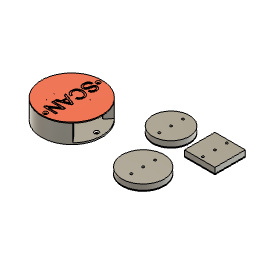
RFID Scanner und Tags (Autodesk Fusion 360 design; units mm, degrees)
Autodesk Fusion 360 part; units mm, degrees
sketch "Skizze1" plane through (0, 0, 0) normal (0, 1, 0) x (1, 0, 0)
  circle A0 centre (43.7248, 41.0876) radius 0.4571
  line L0 (55.1328, 36.6645) -> (55.1937, 36.6061)
  circle A1 centre (43.7248, 48.7056) radius 0.4571
  circle A2 centre (38.6462, 41.0876) radius 0.4571
  circle A3 centre (51.3428, 41.0876) radius 0.4571
  circle A4 centre (53.8821, 48.7056) radius 0.4571
  line L1 (7.4561, 1.7442) -> (7.4561, 59.7525) construction
  line L2 (55.1937, 36.6061) -> (55.2521, 36.6645)
  circle A5 centre (33.8119, 10.4896) radius 0.4571
  circle A6 centre (31.2827, -2.334) radius 0.4571
  circle A7 centre (53.3748, -5.0003) radius 0.4571
  circle A8 centre (20.871, 41.0876) radius 0.4571
  circle A9 centre (53.3748, -2.461) radius 0.4571
  circle A10 centre (47.6614, 7.5694) radius 2.5393
  line L3 (67.4454, 59.7662) -> (7.4454, 59.7754)
  circle A11 centre (48.8035, 18.2338) radius 0.4571
  circle A12 centre (33.5676, 18.2338) radius 0.4571
  circle A13 centre (41.1855, 23.3124) radius 0.4571
  circle A14 centre (43.7248, 23.3124) radius 0.4571
  circle A15 centre (25.9496, 23.3124) radius 0.4571
  circle A16 centre (53.8821, 18.2338) radius 0.4571
  circle A17 centre (41.1855, 18.2338) radius 0.4571
  circle A18 centre (51.3428, 23.3124) radius 0.4571
  circle A19 centre (36.1069, 18.2338) radius 0.4571
  line L4 (55.1937, 36.7229) -> (55.1328, 36.6645)
  line L5 (55.2521, 36.6645) -> (55.1937, 36.7229)
  circle A20 centre (38.7737, 31.8199) radius 0.4571
  circle A21 centre (18.3317, 48.7055) radius 0.4571
  circle A22 centre (23.4103, 18.2338) radius 0.4571
  circle A23 centre (48.8035, 48.7056) radius 0.4571
  circle A24 centre (48.8035, 41.0876) radius 0.4571
  circle A25 centre (46.3917, 7.5694) radius 0.4063
  circle A26 centre (36.1069, 23.3124) radius 0.4571
  circle A27 centre (38.6462, 18.2338) radius 0.4571
  circle A28 centre (31.0282, 23.3124) radius 0.4571
  circle A29 centre (23.4103, 23.3124) radius 0.4571
  circle A30 centre (28.4889, 18.2338) radius 0.4571
  circle A31 centre (33.5676, 48.7071) radius 0.4571
  circle A32 centre (46.2642, 48.7056) radius 0.4571
  circle A33 centre (36.1069, 41.0876) radius 0.4571
  circle A34 centre (15.7923, 41.0876) radius 0.4571
  circle A35 centre (41.1855, 41.0876) radius 0.4571
  circle A36 centre (25.9496, 41.0876) radius 0.4571
  circle A37 centre (51.3428, 48.7056) radius 0.4571
  circle A38 centre (20.871, 48.7056) radius 0.4571
  circle A39 centre (31.0282, 41.0876) radius 0.4571
  circle A40 centre (19.9828, 32.8356) radius 2.5393
  circle A41 centre (18.3317, 41.0876) radius 0.4571
  circle A42 centre (21.2524, 32.8356) radius 0.4063
  circle A43 centre (23.4103, 48.7056) radius 0.4571
  circle A44 centre (28.4889, 41.0891) radius 0.4571
  circle A45 centre (15.7923, 48.7056) radius 0.4571
  circle A46 centre (26.2041, -2.334) radius 0.4571
  circle A47 centre (28.4889, 48.7056) radius 0.4571
  circle A48 centre (48.931, 7.5694) radius 0.4063
  circle A49 centre (53.3748, 0.0784) radius 0.4571
  circle A50 centre (25.9496, 48.7056) radius 0.4571
  circle A51 centre (36.3512, 10.4896) radius 0.4571
  circle A52 centre (31.2726, 10.4896) radius 0.4571
  circle A53 centre (12.4547, 54.7297) radius 1.9995
  circle A54 centre (31.0282, 48.7056) radius 0.4571
  circle A55 centre (18.7131, 32.8356) radius 0.4063
  circle A56 centre (23.4103, 41.0876) radius 0.4571
  circle A57 centre (36.3614, -2.334) radius 0.4571
  circle A58 centre (28.7434, -2.334) radius 0.4571
  circle A59 centre (38.9007, -2.334) radius 0.4571
  circle A60 centre (33.822, -2.334) radius 0.4571
  circle A61 centre (51.3428, 18.2338) radius 0.4571
  circle A62 centre (43.7248, 18.2338) radius 0.4571
  circle A63 centre (25.9496, 18.2338) radius 0.4571
  circle A64 centre (46.2642, 18.2338) radius 0.4571
  circle A65 centre (31.0282, 18.2338) radius 0.4571
  circle A66 centre (48.8035, 23.3124) radius 0.4571
  circle A67 centre (46.2642, 23.3124) radius 0.4571
  circle A68 centre (33.5676, 23.3124) radius 0.4571
  circle A69 centre (28.4889, 23.3124) radius 0.4571
  circle A70 centre (53.8821, 23.3124) radius 0.4571
  circle A71 centre (38.6462, 23.3124) radius 0.4571
  circle A72 centre (38.8905, 10.4896) radius 0.4571
  circle A73 centre (38.6462, 48.7056) radius 0.4571
  line L6 (67.4454, -10.2338) -> (67.4454, 59.7662)
  circle A74 centre (53.8821, 41.0876) radius 0.4571
  circle A75 centre (33.5676, 41.0876) radius 0.4571
  circle A76 centre (41.313, 31.8199) radius 0.4571
  circle A77 centre (41.1855, 48.7056) radius 0.4571
  line L7 (7.4561, -0.2529) -> (7.4561, -10.2529) construction
  line L8 (7.4561, -10.2529) -> (7.4561, 1.7442) construction
  circle A78 centre (12.4553, -5.2434) radius 2
  circle A79 centre (61.5007, 4.2682) radius 0.4571
  circle A80 centre (61.5007, 16.9649) radius 0.4571
  spline S0 degree 3 poles (17.1778, 15.3914) (17.1778, 15.4319) (17.1448, 15.4675) (17.1016, 15.4675) knots 0 0 0 0 1 1 1 1
  circle A81 centre (46.2642, 41.0876) radius 0.4571
  circle A82 centre (18.3422, 18.2345) radius 0.4571
  line L9 (19.1711, 0.8207) -> (19.222, 0.8715)
  line L10 (19.1711, 0.9248) -> (19.1204, 0.8715)
  circle A83 centre (62.4454, -5.2338) radius 2
  circle A84 centre (20.871, 18.2338) radius 0.4571
  circle A85 centre (15.7923, 23.3124) radius 0.4571
  circle A86 centre (15.7928, 18.2345) radius 0.4571
  spline S1 degree 3 poles (17.028, 15.3914) (17.028, 15.3507) (17.061, 15.3151) (17.1016, 15.3151) knots 0 0 0 0 1 1 1 1
  spline S2 degree 3 poles (17.1016, 15.3151) (17.1448, 15.3151) (17.1778, 15.3507) (17.1778, 15.3914) knots 0 0 0 0 1 1 1 1
  circle A87 centre (18.3317, 23.3124) radius 0.4571
  line L11 (19.1204, 0.8715) -> (19.1711, 0.8207)
  spline S3 degree 3 poles (17.1016, 15.4675) (17.061, 15.4675) (17.028, 15.4319) (17.028, 15.3914) knots 0 0 0 0 1 1 1 1
  circle A88 centre (20.871, 23.3124) radius 0.4571
  line L12 (19.222, 0.8715) -> (19.1711, 0.9248)
  circle A89 centre (36.1069, 48.7056) radius 0.4571
  line L13 (7.4546, -10.2338) -> (67.4454, -10.2338)
  circle A90 centre (62.4413, 54.7297) radius 1.9995
  line L14 (7.4454, 59.7754) -> (7.4546, -10.2338)
  line L15 (7.4561, 59.7525) -> (67.4454, -10.2338) construction
  line L16 (67.4454, 59.7662) -> (7.4546, -10.2338) construction
  circle A91 centre (37.0735, 24.204) radius 49.5
  circle A92 centre (37.0735, 24.204) radius 48
  line L17 (37.45, 24.7662) -> (62.4413, 54.7297) construction
  line L18 (62.4413, 54.7297) -> (68.7244, 62.2628) construction
  line L19 (37.45, 24.7662) -> (12.4547, 54.7297) construction
  line L20 (12.4547, 54.7297) -> (5.8664, 62.6275) construction
  line L21 (37.45, 24.7662) -> (12.4553, -5.2434) construction
  line L22 (12.4553, -5.2434) -> (5.3402, -13.7861) construction
  line L23 (37.45, 24.7662) -> (62.4454, -5.2338) construction
  line L24 (62.4454, -5.2338) -> (79.7938, -26.0558) construction
  line L25 (12.4547, 54.7297) -> (0.6399, 44.8739) construction
  line L26 (12.4553, -5.2434) -> (16.2802, -8.429) construction
  line L27 (62.4454, -5.2338) -> (57.9412, -8.9866) construction
  line L28 (15.6414, -5.7932) -> (14.5245, -2.759)
  line L29 (14.5245, -2.759) -> (11.3384, -2.2092)
  line L30 (11.3384, -2.2092) -> (9.2693, -4.6936)
  line L31 (9.2693, -4.6936) -> (10.3862, -7.7277)
  line L32 (10.3862, -7.7277) -> (13.5722, -8.2775)
  line L33 (13.5722, -8.2775) -> (15.6414, -5.7932)
  line L34 (11.3402, 51.6947) -> (14.5258, 52.2469)
  line L35 (14.5258, 52.2469) -> (15.6404, 55.2819)
  line L36 (15.6404, 55.2819) -> (13.5693, 57.7646)
  line L37 (13.5693, 57.7646) -> (10.3837, 57.2124)
  line L38 (10.3837, 57.2124) -> (9.2691, 54.1774)
  line L39 (9.2691, 54.1774) -> (11.3402, 51.6947)
  line L40 (61.329, -8.2681) -> (64.515, -7.7178)
  line L41 (64.515, -7.7178) -> (65.6314, -4.6835)
  line L42 (65.6314, -4.6835) -> (63.5618, -2.1995)
  line L43 (63.5618, -2.1995) -> (60.3758, -2.7498)
  line L44 (60.3758, -2.7498) -> (59.2594, -5.7842)
  line L45 (59.2594, -5.7842) -> (61.329, -8.2681)
  line L46 (65.627, 54.1777) -> (64.5122, 57.2126)
  line L47 (64.5122, 57.2126) -> (61.3265, 57.7646)
  line L48 (61.3265, 57.7646) -> (59.2556, 55.2817)
  line L49 (59.2556, 55.2817) -> (60.3704, 52.2468)
  line L50 (60.3704, 52.2468) -> (63.5561, 51.6948)
  line L51 (63.5561, 51.6948) -> (65.627, 54.1777)
  line L52 (7.4561, 56.3508) -> (7.4458, 56.3631)
  line L53 (59.2594, -5.7842) -> (57.7337, -3.953)
  line L54 (63.5618, -2.1995) -> (62.0361, -0.3684)
  line L55 (59.2556, 55.2817) -> (57.729, 53.4513)
  line L56 (63.5561, 51.6948) -> (62.0295, 49.8644)
  line L57 (15.6404, 55.2819) -> (17.1672, 53.4517)
  line L58 (11.3402, 51.6947) -> (12.8669, 49.8645)
  line L59 (11.3384, -2.2092) -> (12.8638, -0.3779)
  line L60 (15.6414, -5.7932) -> (17.1668, -3.9618)
  line L61 (62.4454, -5.2338) -> (59.8849, -2.1607)
  line L62 (59.8849, -2.1607) -> (56.0435, -5.3613)
  line L63 (56.0435, -5.3613) -> (58.604, -8.4344)
  line L64 (58.604, -8.4344) -> (62.4454, -5.2338)
  line L65 (56.0435, -5.3613) -> (63.7263, 1.0399)
  line L66 (63.7263, 1.0399) -> (72.8923, -9.9613)
  line L67 (65.2939, -16.4637) -> (56.0435, -5.3613)
  line L68 (66.2811, 51.5271) -> (63.719, 48.4553)
  line L69 (63.719, 48.4553) -> (59.8793, 51.6579)
  line L70 (63.719, 48.4553) -> (56.0395, 54.8605)
  line L71 (56.0395, 54.8605) -> (63.719, 48.4553)
  line L72 (63.719, 48.4553) -> (72.4066, 58.8713)
  line L73 (64.7179, 65.2654) -> (56.0395, 54.8605)
  line L74 (8.6153, 51.5268) -> (11.1776, 48.4552)
  line L75 (11.1776, 48.4552) -> (15.017, 51.6581)
  line L76 (15.017, 51.6581) -> (12.4547, 54.7297)
  line L77 (11.1776, 48.4552) -> (18.8565, 54.8609)
  line L78 (18.8565, 54.8609) -> (9.9104, 65.5853)
  line L79 (2.1469, 59.2808) -> (11.1776, 48.4552)
  line L80 (12.4553, -5.2434) -> (16.2973, -8.4433)
  line L81 (16.2973, -8.4433) -> (18.8572, -5.3697)
  line L82 (18.8572, -5.3697) -> (15.0153, -2.1698)
  line L83 (15.0153, -2.1698) -> (12.4553, -5.2434)
  line L84 (18.8572, -5.3697) -> (11.1733, 1.0301)
  line L85 (11.1733, 1.0301) -> (1.6648, -10.3861)
  line L86 (9.3396, -16.797) -> (18.8572, -5.3697)
  line L87 (37.45, 24.7662) -> (37.2153, 73.7038) construction
  line L88 (37.45, 24.7662) -> (-12.4233, 24.7662) construction
  line L89 (37.45, 24.7662) -> (86.5703, 24.7662) construction
  line L90 (37.45, -25.2946) -> (37.45, 24.7662) construction
  circle A93 centre (37.45, -19.0446) radius 2
  circle A94 centre (-3.1733, 24.7662) radius 2
  circle A95 centre (37.2452, 67.4539) radius 2
  circle A96 centre (77.3203, 24.7662) radius 2
  line L91 (13.1402, -12.2338) -> (61.7696, -12.2338)
  line L92 (68.2776, -12.2338) -> (68.3191, -12.2338)
  line L93 (61.8, 61.767) -> (13.0893, 61.7745)
  line L94 (37.45, -19.0446) -> (28.5395, -19.0446) construction
  line L95 (37.2452, 67.4539) -> (27.1977, 67.4057) construction
  line L96 (34.453, 65.8239) -> (37.2608, 64.2207)
  line L97 (37.2608, 64.2207) -> (40.053, 65.8507)
  line L98 (40.053, 65.8507) -> (40.0375, 69.0838)
  line L99 (40.0375, 69.0838) -> (37.2297, 70.687)
  line L100 (37.2297, 70.687) -> (34.4375, 69.057)
  line L101 (34.4375, 69.057) -> (34.453, 65.8239)
  line L102 (34.4835, 69.0838) -> (34.4453, 69.0838)
  line L103 (34.65, -20.6612) -> (37.45, -22.2777)
  line L104 (37.45, -22.2777) -> (40.25, -20.6612)
  line L105 (40.25, -20.6612) -> (40.25, -17.428)
  line L106 (40.25, -17.428) -> (37.45, -15.8114)
  line L107 (37.45, -15.8114) -> (34.65, -17.428)
  line L108 (34.65, -17.428) -> (34.65, -20.6612)
  line L109 (13.0893, 61.7745) -> (37.4447, 61.7708)
  line L110 (13.0893, 61.7745) -> (7.2006, 61.7754)
  line L111 (61.8, 61.767) -> (66.9569, 61.767)
  line L112 (61.7696, -12.2338) -> (68.3191, -12.2338)
  line L113 (13.1402, -12.2338) -> (5.8279, -12.2338)
  line L114 (34.65, -17.428) -> (34.65, -12.2338)
  line L115 (34.65, -12.2338) -> (40.25, -12.2338)
  line L116 (40.25, -12.2338) -> (40.25, -17.428)
  line L117 (34.453, 65.8507) -> (34.453, 61.7712)
  line L118 (40.053, 61.7704) -> (40.053, 65.8507)
  point P0 (10.0297, 9.9978)
  point P1 (10.0296, 9.6931)
  point P2 (37.2005, 32.5977)
  point P3 (37.2004, 32.293)
  point P4 (39.7398, 32.5977)
  point P5 (39.7397, 32.293)
  point P6 (10.8814, -3.2387)
  point P7 (60.868, -3.2387)
  point P8 (10.8814, 56.7452)
  point P9 (12.4553, -5.2434)
  point P10 (9.9026, 3.8046)
  point P11 (62.4454, -5.2338)
  point P12 (12.1959, -5.1606)
  point P13 (37.0735, 24.204)
  point P14 (9.9027, 4.1093)
  point P15 (62.4413, 54.7297)
  point P16 (12.4547, 54.7297)
  point P17 (12.1959, -5.1606)
  point P18 (63.8268, -5.427)
  point P19 (-4.5599, -10.2338)
  point P20 (12.4553, -5.2434)
  point P21 (12.4547, 54.7297)
  point P22 (62.4454, -5.2338)
  point P23 (62.4413, 54.7297)
  point P24 (37.2452, 67.4539)
  point P25 (37.45, -19.0446)
  dimension "d5" = 10
  dimension "d10" = 4
  dimension "d11" = 4
  dimension "d14" = 60
  dimension "d15" = 70
  dimension "d17" = 99
  dimension "d18" = -1.5
  dimension "d19" = 2.8
  dimension "d20" = 2.8
  dimension "d21" = 2.8
  dimension "d22" = 2.8
  dimension "d23" = 5
  dimension "d24" = 10
  dimension "d25" = 5
  dimension "d26" = 4
  dimension "d27" = 10
  dimension "d28" = 5
  dimension "d29" = 4
  dimension "d30" = 10
  dimension "d31" = 4
  dimension "d32" = 5
  dimension "d33" = 10
  dimension "d42" = 4
  dimension "d44" = 4
  dimension "d46" = 4
  dimension "d48" = 4
  dimension "d56" = 2.8
  dimension "d57" = 2.8
  constraint coincident P23 P15
  constraint coincident P17 P12
  constraint vertical L7
  constraint coincident L13.start L14.end
  constraint coincident P20 P9
  constraint coincident P22 P11
  constraint coincident P13 A91.centre
  constraint midpoint L16 L17.start
  constraint parallel L17 L18
  constraint coincident P21 P16
  constraint parallel L19 L20
  constraint parallel L21 L22
  constraint parallel L23 L24
  constraint perpendicular L20 L25
  constraint perpendicular L24 L27
  constraint perpendicular L22 L26
  constraint coincident A91 L18.end
  constraint coincident A91 L20.end
  constraint parallel L39 L52
  constraint coincident A91 L22.end
  constraint perpendicular L61 L62
  constraint parallel L61 L63
  constraint parallel L62 L64
  constraint parallel L23 L61
  constraint perpendicular L65 L66
  constraint parallel L66 L67
  constraint perpendicular L63 L65
  constraint parallel L48 L55
  constraint parallel L51 L56
  constraint parallel L36 L57
  constraint parallel L39 L58
  constraint parallel L30 L59
  constraint parallel L33 L60
  constraint perpendicular L17 L70
  constraint perpendicular L71 L72
  constraint parallel L72 L73
  constraint parallel L74 L76
  constraint perpendicular L77 L78
  constraint parallel L78 L79
  constraint perpendicular L76 L77
  constraint perpendicular L80 L81
  constraint parallel L80 L82
  constraint parallel L81 L83
  constraint parallel L26 L80
  constraint perpendicular L84 L85
  constraint parallel L85 L86
  constraint perpendicular L83 L84
  constraint coincident L84 L59.end
  constraint coincident L82 L60.end
  constraint coincident A91 L85.end
  constraint coincident A91 L86.start
  constraint coincident A91 L79.start
  constraint coincident A91 L78.end
  constraint coincident L77 L57.end
  constraint coincident L75 L58.end
  constraint coincident L14 L52.end
  constraint coincident L1 L52.start
  constraint coincident A91 L67.start
  constraint coincident A91 L66.end
  constraint parallel L42 L54
  constraint parallel L45 L53
  constraint coincident L65 L54.end
  constraint coincident L62 L53.end
  constraint coincident L70 L55.end
  constraint coincident L69 L56.end
  constraint coincident A91 L72.end
  constraint coincident A91 L73.start
  constraint horizontal L88
  constraint horizontal L89
  constraint vertical L90
  constraint coincident A91 L90.start
  constraint coincident A91 L89.end
  constraint coincident A91 L88.end
  constraint coincident A91 L87.end
  constraint coincident L90 P25
  constraint coincident L88 A94.centre
  constraint coincident L87 P24
  constraint coincident L89 A96.centre
  constraint coincident L67 L91.end
  constraint coincident L24 L92.start
  constraint collinear L91 L92
  constraint coincident A92 L92.end
  constraint coincident L73 L93.start
  constraint coincident L78 L93.end
  constraint coincident L86 L91.start
  constraint coincident P25 A93.centre
  constraint perpendicular L90 L94
  constraint coincident P24 A95.centre
  constraint perpendicular L87 L95
  constraint horizontal L102
  constraint coincident L100 L102.start
  constraint parallel L93 L109
  constraint coincident A92 L110.end
  constraint parallel L93 L110
  constraint horizontal L111
  constraint coincident A92 L111.end
  constraint parallel L92 L112
  constraint horizontal L113
  constraint coincident A92 L113.end
  constraint vertical L114
  constraint horizontal L115
  constraint vertical L116
  constraint coincident L91 L114.end
  constraint vertical L117
  constraint vertical L118
  constraint coincident L93 L117.end
  constraint coincident L93 L118.start
  measures "d5" distance of L7.start L7.end
  measures "d10" diameter of A78
  measures "d11" diameter of A83
  measures "d14" distance of L3.end L3.start
  measures "d15" distance of L6.start L3.start
  measures "d17" diameter of A91
  measures "d19" distance of P20 L33
  measures "d20" distance of P21 L39
  measures "d21" distance of P22 L45
  measures "d22" distance of P23 L51
  measures "d23" distance of P22 L63.end
  measures "d24" distance of L62.end L65.end
  measures "d25" distance of P23 L68.start
  measures "d26" distance of P23 L69.end
  measures "d27" distance of L68.end L70.end
  measures "d28" distance of P21 L74.start
  measures "d29" distance of P21 L75.end
  measures "d30" distance of L74.end L77.end
  measures "d31" distance of P20 L82.end
  measures "d32" distance of L81 L83
  measures "d33" distance of L81.end L84.end
  measures "d42" diameter of A93
  measures "d44" diameter of A94
  measures "d46" diameter of A95
  measures "d48" diameter of A96
  measures "d56" distance of P24 L101
  measures "d57" distance of P25 L108
extrude "Extrusion1" add sketch "Skizze1" against normal blind 2.5 contours A0 | A1 | A2 | A3 | A4 | A5 | A6 | A7 | A8 | A9 | A10 | L3 L6 L46 L47 L48 L51 L55 L56 L68 L69 L70 L71 L72 L73 | L3 L6 A92 L72 L73 L111 | L3 L6 L13 L14 L62 L63 L65 L66 L67 L68 L69 L70 L71 L72 L73 L74 L75 L77 L78 L79 L81 L82 L84 L85 L86 | L3 L73 L78 L93 L109 | L6 A92 L66 L72 | L3 L14 L36 L37 L38 L39 L57 L58 L74 L75 L77 L78 L79 | L3 L14 A92 L78 L79 L110 | A92 L73 L78 L93 L98 L99 L100 L101 L109 L117 L118 | A92 L73 L111 | L6 L13 A92 L66 L67 L92 L112 | L6 L13 L40 L41 L42 L45 L54 L64 L65 L66 L67 | A91 A92 L66 L72 | A91 A92 L72 L73 | A92 L78 L110 | A91 A92 L73 L78 | L93 L96 L97 L109 L117 L118 | L49 L50 L55 L56 L69 L70 L71 | A91 A92 L66 L67 | L35 L57 L76 L77 | A91 A92 L78 L79 | L96 L97 L98 L99 L100 L101 L117 | L46 L47 L48 L49 L50 L51 | L13 L67 L86 L91 L115 | L43 L54 L61 L65 | A92 L67 L92 L112 | L14 A92 L79 L85 | L34 L35 L36 L37 L38 L39 | L34 L58 L75 L76 L77 | A91 A92 L79 L85 | L13 L14 A92 L85 L86 L113 | L13 L14 L30 L31 L32 L33 L59 L80 L84 L85 L86 | A92 L67 L86 L91 L103 L104 L105 L108 L114 L116 | L45 L53 L62 L63 L64 L65 L67 | A83 L40 L41 L42 L43 L45 L61 L64 | L44 L53 L61 L62 L65 | A91 A92 L67 L86 | A91 A92 L85 L86 | A92 L86 L113 | L33 L60 L80 L81 L82 L84 L86 | L91 L106 L107 L114 L115 L116 | A83 L44 L45 L61 L64 | A78 L28 L33 L80 L83 | A78 L29 L30 L31 L32 L33 L80 L83 | L103 L104 L105 L106 L107 L108 | A83 L61 L64 | A83 L61 L64 | L29 L59 L83 L84 | L28 L60 L82 L83 L84 | A78 L80 L83 | A78 L80 L83 | A11 | A12 | A13 | A14 | A15 | A16 | A17 | A18 | A19 | A20 | A21 | A22 | A23 | A24 | A25 | A26 | A27 | A28 | A29 | A30 | A31 | A32 | A33 | A34 | A35 | A36 | A37 | A38 | A39 | A40 | A41 | A42 | A43 | A44 | A45 | A46 | A47 | A48 | A49 | A50 | A51 | A52 | A53 | A54 | A55 | A56 | A57 | A58 | A59 | A60 | A61 | A62 | A63 | A64 | A65 | A66 | A67 | A68 | A69 | A70 | A71 | A72 | A73 | A74 | A75 | A76 | A77 | A79 | A80 | A81 | A82 | A84 | A85 | A86 | A87 | A88 | A89 | A90 | A93 | A95 makes body 1
chamfer "Fase2" distance 1.7 angle 45 2 edges at (75.4557, 0, -25.4894) (-5.038, 0, -25.4894) on bodies 1
extrude "Extrusion2" add sketch "Skizze1" along normal blind 19 contours L3 L6 L46 L47 L48 L51 L55 L56 L68 L69 L70 L71 L72 L73 | L3 L6 A92 L72 L73 L111 | L3 L14 L36 L37 L38 L39 L57 L58 L74 L75 L77 L78 L79 | L3 L14 A92 L78 L79 L110 | A92 L73 L111 | L6 L13 A92 L66 L67 L92 L112 | L6 L13 L40 L41 L42 L45 L54 L64 L65 L66 L67 | A91 A92 L72 L73 | A92 L78 L110 | L49 L50 L55 L56 L69 L70 L71 | A91 A92 L66 L67 | L35 L57 L76 L77 | L46 L47 L48 L49 L50 L51 | L43 L54 L61 L65 | A92 L67 L92 L112 | L34 L35 L36 L37 L38 L39 | L34 L58 L75 L76 L77 | L13 L14 A92 L85 L86 L113 | L13 L14 L30 L31 L32 L33 L59 L80 L84 L85 L86 | L45 L53 L62 L63 L64 L65 L67 | A83 L40 L41 L42 L43 L45 L61 L64 | L44 L53 L61 L62 L65 | A91 A92 L85 L86 | A92 L86 L113 | L33 L60 L80 L81 L82 L84 L86 | A83 L44 L45 L61 L64 | A78 L28 L33 L80 L83 | A78 L29 L30 L31 L32 L33 L80 L83 | L29 L59 L83 L84 | L28 L60 L82 L83 L84 bodies 1
extrude "Extrusion3" cut sketch "Skizze1" against normal blind 2.5 from surface at 17.5 contours L49 L50 L55 L56 L69 L70 L71 | L35 L57 L76 L77 | L46 L47 L48 L49 L50 L51 | L43 L54 L61 L65 | L34 L35 L36 L37 L38 L39 | L34 L58 L75 L76 L77 | A83 L40 L41 L42 L43 L45 L61 L64 | L44 L53 L61 L62 L65 | A83 L44 L45 L61 L64 | A78 L28 L33 L80 L83 | A78 L29 L30 L31 L32 L33 L80 L83 | A83 L61 L64 | A83 L61 L64 | L29 L59 L83 L84 | L28 L60 L82 L83 L84 | A78 L80 L83 | A78 L80 L83 | A53 | A90 bodies 1
extrude "Extrusion4" add sketch "Skizze1" along normal blind 28 contours A92 L73 L78 L93 L98 L99 L100 L101 L109 L117 L118 | A92 L73 L111 | A91 A92 L72 L73 | A92 L78 L110 | A91 A92 L73 L78 | L93 L96 L97 L109 L117 L118 | A91 A92 L66 L67 | A91 A92 L78 L79 | L96 L97 L98 L99 L100 L101 L117 | A92 L67 L92 L112 | A92 L67 L86 L91 L103 L104 L105 L108 L114 L116 | A91 A92 L67 L86 | A91 A92 L85 L86 | A92 L86 L113 | L91 L106 L107 L114 L115 L116 | L103 L104 L105 L106 L107 L108 | A93 | A95 bodies 1
extrude "Extrusion5" cut sketch "Skizze1" against normal blind 2.5 from surface at 26.5 contours L93 L96 L97 L109 L117 L118 | L96 L97 L98 L99 L100 L101 L117 | L91 L106 L107 L114 L115 L116 | L103 L104 L105 L106 L107 L108 | A93 | A95 bodies 1
extrude "Extrusion6" cut sketch "Skizze1" along normal blind 26.5 from surface at 1.5 contours A93 | A95 bodies 1
fillet "Abrundung1" radius 7 8 edges at (61.7696, 9.5, 12.2338) (13.1402, 9.5, 12.2338) (61.8, 9.5, -61.767) (13.0893, 9.5, -61.7745) (66.9569, 23.5, -61.767) (7.2006, 23.5, -61.7754) (5.8279, 23.5, 12.2338) (68.3191, 23.5, 12.2338) on bodies 1
extrude "Extrusion7" add sketch "Skizze1" along normal blind 1.5 from surface at 28 separate body contours A0 | A1 | A2 | A3 | A4 | A5 | A6 | A7 | A8 | A9 | A10 | L3 L6 L46 L47 L48 L51 L55 L56 L68 L69 L70 L71 L72 L73 | L3 L6 A92 L72 L73 L111 | L3 L6 L13 L14 L62 L63 L65 L66 L67 L68 L69 L70 L71 L72 L73 L74 L75 L77 L78 L79 L81 L82 L84 L85 L86 | L3 L73 L78 L93 L109 | L6 A92 L66 L72 | L3 L14 L36 L37 L38 L39 L57 L58 L74 L75 L77 L78 L79 | L3 L14 A92 L78 L79 L110 | A92 L73 L78 L93 L98 L99 L100 L101 L109 L117 L118 | A92 L73 L111 | L6 L13 A92 L66 L67 L92 L112 | L6 L13 L40 L41 L42 L45 L54 L64 L65 L66 L67 | A91 A92 L66 L72 | A91 A92 L72 L73 | A92 L78 L110 | A91 A92 L73 L78 | L93 L96 L97 L109 L117 L118 | L49 L50 L55 L56 L69 L70 L71 | A91 A92 L66 L67 | L35 L57 L76 L77 | A91 A92 L78 L79 | L96 L97 L98 L99 L100 L101 L117 | L46 L47 L48 L49 L50 L51 | L13 L67 L86 L91 L115 | L43 L54 L61 L65 | A92 L67 L92 L112 | L14 A92 L79 L85 | L34 L35 L36 L37 L38 L39 | L34 L58 L75 L76 L77 | A91 A92 L79 L85 | L13 L14 A92 L85 L86 L113 | L13 L14 L30 L31 L32 L33 L59 L80 L84 L85 L86 | A92 L67 L86 L91 L103 L104 L105 L108 L114 L116 | L45 L53 L62 L63 L64 L65 L67 | A83 L40 L41 L42 L43 L45 L61 L64 | L44 L53 L61 L62 L65 | A91 A92 L67 L86 | A91 A92 L85 L86 | A92 L86 L113 | L33 L60 L80 L81 L82 L84 L86 | L91 L106 L107 L114 L115 L116 | A83 L44 L45 L61 L64 | A78 L28 L33 L80 L83 | A78 L29 L30 L31 L32 L33 L80 L83 | L103 L104 L105 L106 L107 L108 | A83 L61 L64 | A83 L61 L64 | L29 L59 L83 L84 | L28 L60 L82 L83 L84 | A78 L80 L83 | A78 L80 L83 | A11 | A12 | A13 | A14 | A15 | A16 | A17 | A18 | A19 | A20 | A21 | A22 | A23 | A24 | A25 | A26 | A27 | A28 | A29 | A30 | A31 | A32 | A33 | A34 | A35 | A36 | A37 | A38 | A39 | A40 | A41 | A42 | A43 | A44 | A45 | A46 | A47 | A48 | A49 | A50 | A51 | A52 | A53 | A54 | A55 | A56 | A57 | A58 | A59 | A60 | A61 | A62 | A63 | A64 | A65 | A66 | A67 | A68 | A69 | A70 | A71 | A72 | A73 | A74 | A75 | A76 | A77 | A79 | A80 | A81 | A82 | A84 | A85 | A86 | A87 | A88 | A89 | A90 | A94 | A96 makes body 2
chamfer "Fase1" distance 1.5 angle 45 2 edges at (35.3806, 29.5, -68.1771) (35.5853, 29.5, 18.3213) on bodies 2
sketch "Skizze2" plane through (0, 29.5, 0) normal (0, 1, 0) x (-1, 0, 0)
  circle A0 centre (-37.2452, -67.4539) radius 3.5
  line L0 (-19.1711, -0.9248) -> (-19.222, -0.8715)
  line L1 (-19.222, -0.8715) -> (-19.1711, -0.8207)
  line L2 (-19.1711, -0.8207) -> (-19.1204, -0.8715)
  line L3 (-19.1204, -0.8715) -> (-19.1711, -0.9248)
  line L4 (-55.1937, -36.7229) -> (-55.2521, -36.6645)
  line L5 (-55.2521, -36.6645) -> (-55.1937, -36.6061)
  line L6 (-55.1937, -36.6061) -> (-55.1328, -36.6645)
  line L7 (-55.1328, -36.6645) -> (-55.1937, -36.7229)
  spline S0 degree 3 poles (-17.028, -15.3914) (-17.028, -15.4319) (-17.061, -15.4675) (-17.1016, -15.4675) knots -1 -1 -1 -1 0 0 0 0
  spline S1 degree 3 poles (-17.1016, -15.4675) (-17.1448, -15.4675) (-17.1778, -15.4319) (-17.1778, -15.3914) knots -1 -1 -1 -1 0 0 0 0
  spline S2 degree 3 poles (-17.1778, -15.3914) (-17.1778, -15.3507) (-17.1448, -15.3151) (-17.1016, -15.3151) knots -1 -1 -1 -1 0 0 0 0
  spline S3 degree 3 poles (-17.1016, -15.3151) (-17.061, -15.3151) (-17.028, -15.3507) (-17.028, -15.3914) knots -1 -1 -1 -1 0 0 0 0
  circle A1 centre (-37.0735, -24.204) radius 49.5
  circle A2 centre (-37.45, 19.0446) radius 3.5
  line L8 (-16.1133, -65.5837) -> (-16.1133, 15.2986) construction
  line L9 (-16.1133, 15.2986) -> (-58.0092, 15.2986) construction
  line L10 (-58.0092, 15.2986) -> (-58.0092, -65.5837) construction
  line L11 (-58.0092, -65.5837) -> (-16.1133, -65.5837) construction
  dimension "d79" = 20
  text T0 "SCAN" font "Arial" height 20 align centre middle in box 80.8824 x 41.8959 at (-16.1133, -65.5837) x (0, 1) y (-1, 0) spacing 1 kerned
extrude "Extrusion8" cut sketch "Skizze2" against normal blind 0.7 text T0 bodies 2
sketch "Skizze3" plane through (0, 0, 0) normal (0, 1, 0) x (1, 0, 0)
  circle A0 centre (173.9595, 4.7233) radius 34.5
  circle A1 centre (138.5672, 85.9638) radius 30
  line L0 (233.7071, 112.8918) -> (183.7071, 112.8918)
  line L1 (183.7071, 112.8918) -> (183.7071, 62.8918)
  line L2 (183.7071, 62.8918) -> (233.7071, 62.8918)
  line L3 (233.7071, 62.8918) -> (233.7071, 112.8918)
  line L4 (233.7071, 112.8918) -> (183.7071, 62.8918) construction
  line L5 (183.7071, 112.8918) -> (233.7071, 62.8918) construction
  line L6 (217.2071, 71.8918) -> (200.2071, 71.8918)
  line L7 (188.2071, 83.8918) -> (188.2071, 91.8918)
  line L8 (200.2071, 103.8918) -> (217.2071, 103.8918)
  line L9 (229.2071, 91.8918) -> (229.2071, 83.8918)
  line L10 (229.2071, 71.8918) -> (188.2071, 103.8918) construction
  line L11 (188.2071, 71.8918) -> (229.2071, 103.8918) construction
  arc A2 (200.2071, 103.8918) -> (188.2071, 91.8918) centre (200.2071, 91.8918) ccw
  arc A3 (188.2071, 83.8918) -> (200.2071, 71.8918) centre (200.2071, 83.8918) ccw
  arc A4 (217.2071, 71.8918) -> (229.2071, 83.8918) centre (217.2071, 83.8918) ccw
  arc A5 (229.2071, 91.8918) -> (217.2071, 103.8918) centre (217.2071, 91.8918) ccw
  line L12 (147.0672, 69.9638) -> (130.0672, 69.9638)
  line L13 (118.0672, 81.9638) -> (118.0672, 89.9638)
  line L14 (130.0672, 101.9638) -> (147.0672, 101.9638)
  line L15 (159.0672, 89.9638) -> (159.0672, 81.9638)
  line L16 (159.0672, 69.9638) -> (118.0672, 101.9638) construction
  line L17 (118.0672, 69.9638) -> (159.0672, 101.9638) construction
  arc A6 (130.0672, 101.9638) -> (118.0672, 89.9638) centre (130.0672, 89.9638) ccw
  arc A7 (159.0672, 89.9638) -> (147.0672, 101.9638) centre (147.0672, 89.9638) ccw
  arc A8 (147.0672, 69.9638) -> (159.0672, 81.9638) centre (147.0672, 81.9638) ccw
  arc A9 (118.0672, 81.9638) -> (130.0672, 69.9638) centre (130.0672, 81.9638) ccw
  line L18 (182.4595, 20.7233) -> (165.4595, 20.7233)
  line L19 (153.4595, 8.7233) -> (153.4595, 0.7233)
  line L20 (165.4595, -11.2767) -> (182.4595, -11.2767)
  line L21 (194.4595, 0.7233) -> (194.4595, 8.7233)
  line L22 (194.4595, 20.7233) -> (153.4595, -11.2767) construction
  line L23 (153.4595, 20.7233) -> (194.4595, -11.2767) construction
  arc A10 (165.4595, 20.7233) -> (153.4595, 8.7233) centre (165.4595, 8.7233) ccw
  arc A11 (194.4595, 8.7233) -> (182.4595, 20.7233) centre (182.4595, 8.7233) ccw
  arc A12 (182.4595, -11.2767) -> (194.4595, 0.7233) centre (182.4595, 0.7233) ccw
  arc A13 (153.4595, 0.7233) -> (165.4595, -11.2767) centre (165.4595, 0.7233) ccw
  line L24 (173.9595, 39.2233) -> (173.9595, -29.7767) construction
  line L25 (208.7071, 122.5963) -> (208.7071, 48.5117) construction
  line L26 (138.5672, 115.9638) -> (138.5672, 55.9638) construction
  circle A14 centre (173.9595, 20.7233) radius 3.5 construction
  circle A15 centre (173.9595, 24.2233) radius 1.85
  line L27 (173.9595, 24.2233) -> (181.1537, 24.2233) construction
  line L28 (176.7595, 25.8399) -> (173.9595, 27.4564)
  line L29 (173.9595, 27.4564) -> (171.1595, 25.8399)
  line L30 (171.1595, 25.8399) -> (171.1595, 22.6067)
  line L31 (171.1595, 22.6067) -> (173.9595, 20.9901)
  line L32 (173.9595, 20.9901) -> (176.7595, 22.6067)
  line L33 (176.7595, 22.6067) -> (176.7595, 25.8399)
  line L34 (176.7595, 22.6067) -> (176.7595, 20.7233)
  line L35 (176.7595, 20.7233) -> (171.1595, 20.7233)
  line L36 (171.1595, 20.7233) -> (171.1595, 22.6067)
  circle A16 centre (173.9595, -11.2767) radius 3.5 construction
  circle A17 centre (173.9595, -14.7767) radius 1.85
  line L37 (173.9595, -14.7767) -> (180.2552, -14.7767) construction
  line L38 (176.7595, -13.1601) -> (173.9595, -11.5436)
  line L39 (173.9595, -11.5436) -> (171.1595, -13.1601)
  line L40 (171.1595, -13.1601) -> (171.1595, -16.3933)
  line L41 (171.1595, -16.3933) -> (173.9595, -18.0099)
  line L42 (173.9595, -18.0099) -> (176.7595, -16.3933)
  line L43 (176.7595, -16.3933) -> (176.7595, -13.1601)
  line L44 (176.7595, -12.1601) -> (176.7595, -11.2767)
  line L45 (176.7595, -11.2767) -> (171.1595, -11.2767)
  line L46 (171.1595, -11.2767) -> (171.1595, -13.1601)
  circle A18 centre (138.5672, 101.9638) radius 3.5 construction
  circle A19 centre (138.5672, 105.4638) radius 1.85
  line L47 (138.5672, 105.4638) -> (143.9171, 105.4638) construction
  line L48 (141.3672, 107.0804) -> (138.5672, 108.697)
  line L49 (138.5672, 108.697) -> (135.7672, 107.0804)
  line L50 (135.7672, 107.0804) -> (135.7672, 103.8472)
  line L51 (135.7672, 103.8472) -> (138.5672, 102.2306)
  line L52 (138.5672, 102.2306) -> (141.3672, 103.8472)
  line L53 (141.3672, 103.8472) -> (141.3672, 107.0804)
  line L54 (141.3672, 102.8472) -> (141.3672, 101.9638)
  line L55 (141.3672, 101.9638) -> (135.7672, 101.9638)
  line L56 (135.7672, 101.9638) -> (135.7672, 103.8472)
  circle A20 centre (138.5672, 69.9638) radius 3.5 construction
  circle A21 centre (138.5672, 66.4638) radius 1.85
  line L57 (138.5672, 66.4638) -> (145.2484, 66.4638) construction
  line L58 (141.3672, 68.0804) -> (138.5672, 69.697)
  line L59 (138.5672, 69.697) -> (135.7672, 68.0804)
  line L60 (135.7672, 68.0804) -> (135.7672, 64.8472)
  line L61 (135.7672, 64.8472) -> (138.5672, 63.2306)
  line L62 (138.5672, 63.2306) -> (141.3672, 64.8472)
  line L63 (141.3672, 64.8472) -> (141.3672, 68.0804)
  line L64 (141.3672, 68.0804) -> (141.3672, 69.9638)
  line L65 (141.3672, 69.9638) -> (135.7672, 69.9638)
  line L66 (135.7672, 69.9638) -> (135.7672, 68.0804)
  circle A22 centre (208.7071, 103.8918) radius 3.5 construction
  circle A23 centre (208.7071, 71.8918) radius 3.5 construction
  circle A24 centre (208.7071, 107.3918) radius 1.85
  line L67 (208.7071, 107.3918) -> (216.6416, 107.3918) construction
  line L68 (211.5071, 109.0084) -> (208.7071, 110.6249)
  line L69 (208.7071, 110.6249) -> (205.9071, 109.0084)
  line L70 (205.9071, 109.0084) -> (205.9071, 105.7752)
  line L71 (205.9071, 105.7752) -> (208.7071, 104.1586)
  line L72 (208.7071, 104.1586) -> (211.5071, 105.7752)
  line L73 (211.5071, 105.7752) -> (211.5071, 109.0084)
  line L74 (211.5071, 104.7752) -> (211.5071, 103.8918)
  line L75 (211.5071, 103.8918) -> (205.9071, 103.8918)
  line L76 (205.9071, 103.8918) -> (205.9071, 105.7752)
  circle A25 centre (208.7071, 68.3918) radius 1.85
  line L77 (208.7071, 68.3918) -> (217.5709, 68.3918) construction
  line L78 (211.5071, 70.0084) -> (208.7071, 71.6249)
  line L79 (208.7071, 71.6249) -> (205.9071, 70.0084)
  line L80 (205.9071, 70.0084) -> (205.9071, 66.7752)
  line L81 (205.9071, 66.7752) -> (208.7071, 65.1586)
  line L82 (208.7071, 65.1586) -> (211.5071, 66.7752)
  line L83 (211.5071, 66.7752) -> (211.5071, 70.0084)
  line L84 (211.5071, 70.0084) -> (211.5071, 71.8918)
  line L85 (211.5071, 71.8918) -> (205.9071, 71.8918)
  line L86 (205.9071, 71.8918) -> (205.9071, 70.0084)
  circle A26 centre (173.9595, 4.7233) radius 1.85
  circle A27 centre (208.7071, 87.8918) radius 1.85
  circle A28 centre (138.5672, 85.9638) radius 1.85
  point P0 (208.7071, 87.8918)
  point P1 (208.7071, 87.8918)
  point P2 (138.5672, 85.9638)
  point P3 (173.9595, 4.7233)
  point P4 (173.9595, 24.2233)
  point P5 (173.9595, -14.7767)
  point P6 (138.5672, 105.4638)
  point P7 (138.5672, 66.4638)
  point P8 (208.7071, 107.3918)
  point P9 (208.7071, 68.3918)
  dimension "d83" = 69
  dimension "d84" = 60
  dimension "d85" = 50
  dimension "d86" = 50
  dimension "d87" = 41
  dimension "d88" = 32
  dimension "d89" = 12
  dimension "d90" = 41
  dimension "d91" = 32
  dimension "d92" = 12
  dimension "d93" = 41
  dimension "d94" = 32
  dimension "d95" = 12
  dimension "d96" = 7
  dimension "d97" = 3.7
  dimension "d98" = 2.8
  dimension "d99" = 7
  dimension "d100" = 3.7
  dimension "d101" = 2.8
  dimension "d102" = 7
  dimension "d103" = 3.7
  dimension "d104" = 2.8
  dimension "d105" = 7
  dimension "d106" = 3.7
  dimension "d107" = 2.8
  dimension "d108" = 7
  dimension "d109" = 7
  dimension "d110" = 3.7
  dimension "d111" = 2.8
  dimension "d112" = 3.7
  dimension "d113" = 2.8
  dimension "d114" = 3.7
  dimension "d115" = 3.7
  dimension "d116" = 3.7
  constraint horizontal L0
  constraint perpendicular L0 L1
  constraint parallel L0 L2
  constraint parallel L1 L3
  constraint coincident L4 P1
  constraint coincident L5 P1
  constraint horizontal L6
  constraint perpendicular L6 L7
  constraint parallel L6 L8
  constraint parallel L7 L9
  constraint coincident L10 P1
  constraint coincident L11 P1
  constraint coincident P1 P0
  constraint coincident L10.end L8
  constraint coincident L10.end L7
  constraint tangent L8 A2
  constraint tangent L7 A2
  constraint coincident L11.start L6
  constraint coincident L11.start L7
  constraint tangent L6 A3
  constraint tangent L7 A3
  constraint equal A2 A3
  constraint coincident L10.start L9
  constraint coincident L10.start L6
  constraint tangent L9 A4
  constraint tangent L6 A4
  constraint equal A2 A4
  constraint coincident L11.end L8
  constraint coincident L11.end L9
  constraint tangent L8 A5
  constraint tangent L9 A5
  constraint equal A2 A5
  constraint horizontal L12
  constraint perpendicular L12 L13
  constraint parallel L12 L14
  constraint parallel L13 L15
  constraint coincident L16 P2
  constraint coincident L17 P2
  constraint coincident A1.centre A28.centre
  constraint coincident L16.end L13
  constraint coincident L16.end L14
  constraint tangent L13 A6
  constraint tangent L14 A6
  constraint coincident L17.end L15
  constraint coincident L17.end L14
  constraint tangent L15 A7
  constraint tangent L14 A7
  constraint equal A6 A7
  constraint coincident L16.start L12
  constraint coincident L16.start L15
  constraint tangent L12 A8
  constraint tangent L15 A8
  constraint equal A6 A8
  constraint coincident L17.start L13
  constraint coincident L17.start L12
  constraint tangent L13 A9
  constraint tangent L12 A9
  constraint equal A6 A9
  constraint horizontal L18
  constraint perpendicular L18 L19
  constraint parallel L18 L20
  constraint parallel L19 L21
  constraint coincident L22 P3
  constraint coincident L23 P3
  constraint coincident P3 A0.centre
  constraint coincident L23.start L19
  constraint coincident L23.start L18
  constraint tangent L19 A10
  constraint tangent L18 A10
  constraint coincident L22.start L21
  constraint coincident L22.start L18
  constraint tangent L21 A11
  constraint tangent L18 A11
  constraint equal A10 A11
  constraint coincident L23.end L20
  constraint coincident L23.end L21
  constraint tangent L20 A12
  constraint tangent L21 A12
  constraint equal A10 A12
  constraint coincident L22.end L19
  constraint coincident L22.end L20
  constraint tangent L19 A13
  constraint tangent L20 A13
  constraint equal A10 A13
  constraint coincident A0 L24.start
  constraint coincident A0 L24.end
  constraint perpendicular L6 L25
  constraint perpendicular L12 L26
  constraint coincident A1 L26.start
  constraint coincident A1 L26.end
  constraint midpoint L18 A14.centre
  constraint coincident A14 P4
  constraint coincident L24 P4
  constraint coincident P4 A15.centre
  constraint tangent A14 L27
  constraint perpendicular L24 L27
  constraint vertical L34
  constraint horizontal L35
  constraint vertical L36
  constraint coincident L18 L34.end
  constraint midpoint L20 A16.centre
  constraint coincident A16 P5
  constraint coincident L24 P5
  constraint coincident P5 A17.centre
  constraint tangent A16 L37
  constraint perpendicular L24 L37
  constraint vertical L44
  constraint horizontal L45
  constraint vertical L46
  constraint coincident L20 L44.end
  constraint midpoint L14 A18.centre
  constraint coincident A18 P6
  constraint coincident L26 P6
  constraint coincident P6 A19.centre
  constraint tangent A18 L47
  constraint perpendicular L26 L47
  constraint vertical L54
  constraint horizontal L55
  constraint vertical L56
  constraint coincident L14 L54.end
  constraint midpoint L12 A20.centre
  constraint coincident A20 P7
  constraint coincident L26 P7
  constraint coincident P7 A21.centre
  constraint tangent A20 L57
  constraint perpendicular L26 L57
  constraint vertical L64
  constraint horizontal L65
  constraint vertical L66
  constraint coincident L12 L64.end
  constraint midpoint L8 A22.centre
  constraint midpoint L6 A23.centre
  constraint coincident A22 P8
  constraint coincident L25 P8
  constraint coincident P8 A24.centre
  constraint tangent A22 L67
  constraint perpendicular L25 L67
  constraint vertical L74
  constraint horizontal L75
  constraint vertical L76
  constraint coincident L8 L74.end
  constraint coincident A23 P9
  constraint coincident L25 P9
  constraint coincident P9 A25.centre
  constraint tangent A23 L77
  constraint perpendicular L25 L77
  constraint vertical L84
  constraint horizontal L85
  constraint vertical L86
  constraint coincident L6 L84.end
  constraint concentric A1 A28
  measures "d83" diameter of A0
  measures "d84" diameter of A1
  measures "d85" distance of L1.end L2.end
  measures "d86" distance of L0.end L1.end
  measures "d87" distance of L10.end L11.end
  measures "d88" distance of L11.start L10.end
  measures "d89" radius of A2
  measures "d90" distance of L16.end L17.end
  measures "d91" distance of L17.start L16.end
  measures "d92" radius of A6
  measures "d93" distance of L22.end L23.end
  measures "d94" distance of L23.start L22.end
  measures "d95" radius of A10
  measures "d96" diameter of A14
  measures "d97" diameter of A15
  measures "d98" distance of P4 L33
  measures "d99" diameter of A16
  measures "d100" diameter of A17
  measures "d101" distance of P5 L43
  measures "d102" diameter of A18
  measures "d103" diameter of A19
  measures "d104" distance of P6 L53
  measures "d105" diameter of A20
  measures "d106" diameter of A21
  measures "d107" distance of P7 L63
  measures "d108" diameter of A22
  measures "d109" diameter of A23
  measures "d110" diameter of A24
  measures "d111" distance of P8 L73
  measures "d112" diameter of A25
  measures "d113" distance of P9 L83
  measures "d114" diameter of A26
  measures "d115" diameter of A27
  measures "d116" diameter of A28
extrude "Extrusion9" add sketch "Skizze3" along normal blind 9 separate body contours A0 | A1 | L0 L1 L2 L3 | L6 L7 L8 L9 A2 A3 A4 A5 L75 L85 | L6 L78 L79 L84 L85 L86 | L78 L79 L80 L81 L82 L83 | L12 L13 L14 L15 A6 A7 A8 A9 L55 L65 | L12 L58 L59 L64 L65 L66 | L58 L59 L60 L61 L62 L63 | L18 L19 L20 L21 A10 A11 A12 A13 L35 L45 | L18 L31 L32 L34 L35 L36 | L28 L29 L30 L31 L32 L33 | L38 L39 L40 L41 L42 L43 | L48 L49 L50 L51 L52 L53 | L68 L69 L70 L71 L72 L73 makes body 3 at (225.9905, 0, -87.8918) makes body 4 at (163.4387, 0, -17.7015) makes body 5 at (147.8486, 0, -73.8306)
extrude "Extrusion10" cut sketch "Skizze3" along normal blind 4 contours L6 L7 L8 L9 A2 A3 A4 A5 L75 L85 | L12 L13 L14 L15 A6 A7 A8 A9 L55 L65 | L18 L19 L20 L21 A10 A11 A12 A13 L35 L45 bodies 3 4 5
extrude "Extrusion11" cut sketch "Skizze3" along normal blind 2.5 from surface at 1.5 contours L6 L78 L79 L84 L85 L86 | L78 L79 L80 L81 L82 L83 | L12 L58 L59 L64 L65 L66 | L58 L59 L60 L61 L62 L63 | L18 L31 L32 L34 L35 L36 | L28 L29 L30 L31 L32 L33 | A15 | A17 | L38 L39 L40 L41 L42 L43 | A19 | L48 L49 L50 L51 L52 L53 | A21 | L68 L69 L70 L71 L72 L73 | A25 bodies 3 4 5
chamfer "Fase3" distance 1.8 angle 45 3 edges at (206.9823, 4, -88.5608) (136.8424, 4, -86.6328) (172.2347, 4, -5.3923) on bodies 3 4 5
sketch "Skizze4" plane through (0, 0, 0) normal (0, 1, 0) x (1, 0, 0)
  circle A0 centre (138.5672, 66.4638) radius 1.85
  circle A1 centre (138.5672, 105.4638) radius 1.85
  circle A2 centre (138.5672, 85.9638) radius 30
  circle A3 centre (208.7071, 68.3918) radius 1.85
  circle A4 centre (208.7071, 107.3918) radius 1.85
  line L0 (233.7071, 112.8918) -> (233.7071, 62.8918)
  line L1 (233.7071, 62.8918) -> (183.7071, 62.8918)
  line L2 (183.7071, 62.8918) -> (183.7071, 112.8918)
  line L3 (183.7071, 112.8918) -> (233.7071, 112.8918)
  circle A5 centre (173.9595, -14.7767) radius 1.85
  circle A6 centre (173.9595, 24.2233) radius 1.85
  circle A7 centre (173.9595, 4.7233) radius 34.5
  line L4 (234.2214, 97.3643) -> (198.8661, 62.0089) construction
  line L5 (198.8661, 62.0089) -> (183.1929, 77.6821) construction
  line L6 (183.1929, 77.6821) -> (218.5482, 113.0375) construction
  line L7 (218.5482, 113.0375) -> (234.2214, 97.3643) construction
  line L8 (163.0149, 74.8913) -> (113.0149, 74.8913) construction
  line L9 (113.0149, 74.8913) -> (113.0149, 97.0566) construction
  line L10 (113.0149, 97.0566) -> (163.0149, 97.0566) construction
  line L11 (163.0149, 97.0566) -> (163.0149, 74.8913) construction
  line L12 (197.9046, -5.1498) -> (147.9046, -5.1498) construction
  line L13 (147.9046, -5.1498) -> (147.9046, 17.0154) construction
  line L14 (147.9046, 17.0154) -> (197.9046, 17.0154) construction
  line L15 (197.9046, 17.0154) -> (197.9046, -5.1498) construction
  dimension "d127" = 7
  dimension "d128" = 7
  dimension "d129" = 7
  text T0 "Energiepark" font "Arial" height 7 align centre middle in box 50 x 22.1652 at (234.2214, 97.3643) x (-0.707107, -0.707107) y (-0.707107, 0.707107) spacing 1 kerned
  text T1 "Energiepark" font "Arial" height 7 align centre middle in box 50 x 22.1652 at (163.0149, 74.8913) x (-1, 0) y (0, 1) spacing 1 kerned
  text T2 "Energiepark" font "Arial" height 7 align centre middle in box 50 x 22.1652 at (197.9046, -5.1498) x (-1, 0) y (0, 1) spacing 1 kerned
extrude "Extrusion12" add sketch "Skizze4" against normal blind 1.4 separate body makes body 6 at (161.8428, 0, -4.7233) makes body 7 at (191.5884, 0, -93.9723) makes body 8 at (127.9506, 0, -85.9638)
chamfer "Fase4" distance 1.4 angle 45 6 edges at (136.8424, -1.4, -104.7948) (136.8424, -1.4, -65.7948) (206.9823, -1.4, -106.7228) (206.9823, -1.4, -67.7228) (172.2347, -1.4, -23.5543) (172.2347, -1.4, 15.4457) on bodies 6 7 8
extrude "Extrusion13" cut sketch "Skizze4" against normal blind 2 from surface at -0.7 text T1 T2 T0 bodies 6 7 8
